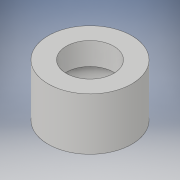
# Autodesk Inventor part: Motor_Magnet_Mount
Saved by Autodesk Inventor 2019 (Build 230136000, 136)
## iProperties
Created: 2019-09-30
Part Number: Motor_Magnet_Mount
Material: Generic
Document SubType Name: Modeling
Designer: isaac
Density: 1 g/cm^3
Appearance: Default
Author: isaac
Autodesk Inventor part; units mm, degrees
ref_plane "YZ Plane" through (0, 0, 0) normal (1, 0, 0) x (0, 1, 0)
ref_plane "XZ Plane" through (0, 0, 0) normal (0, 1, 0) x (-1, 0, 0)
ref_plane "XY Plane" through (0, 0, 0) normal (0, 0, 1) x (1, 0, 0)
sketch "Sketch1" plane through (0, 0, 0) normal (0, 1, 0) x (-1, 0, 0)
  circle A0 centre (0, 0) radius 4.585
  circle A1 centre (0, 0) radius 5.75
  dimension "d0" = 9.17
  dimension "d1" = 11.5
  constraints: 2 centre point, 2 coincident
  measures "d0" diameter of A0
  measures "d1" diameter of A1
extrude "Extrusion1" add sketch "Sketch1" along normal blind 4.1
sketch "Sketch2" plane through (0, 4.1, 0) normal (0, 1, 0) x (1, 0, 0)
  circle A0 centre (0, 0) radius 5.75
  circle A1 centre (0, 0) radius 3.26
  dimension "d4" = 6.52
  dimension "d7" = 11.5
  constraints: 2 centre point, 2 coincident
  measures "d4" diameter of A1
  measures "d7" diameter of A0
extrude "Extrusion2" add sketch "Sketch2" along normal blind 3.1
body "Solid1"
